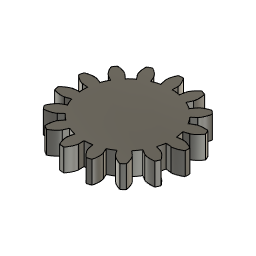
GearTrain v2 (Autodesk Fusion 360 archive; units mm, degrees)
design "15T Mod 2 Gear Base"
Autodesk Fusion 360 part; units mm, degrees
(part 1 of 2)
sketch "Sketch1" plane through (0, 0, 0) normal (0, 0, 1) x (1, 0, 0) in component "Component"
  spline S0 degree 5 poles (13.996, -1.6823) (13.9961, -1.6823) (13.9965, -1.6823) (13.9971, -1.6824) (13.998, -1.6825) (13.9993, -1.6826) (14.0009, -1.6828) (14.0027, -1.6829) (14.0047, -1.6831) (14.0069, -1.6833) (14.0093, -1.6834) (14.0119, -1.6836) (14.0147, -1.6838) (14.0177, -1.684) (14.0209, -1.6842) (14.0242, -1.6844) (14.0278, -1.6846) (14.0315, -1.6848) (14.0354, -1.6849) (14.0394, -1.6851) (14.0436, -1.6853) (14.048, -1.6854) (14.0525, -1.6856) (14.0572, -1.6857) (14.0621, -1.6858) (14.0671, -1.6859) (14.0723, -1.686) (14.0776, -1.6861) (14.083, -1.6861) (14.0886, -1.6861) (14.0944, -1.6862) (14.1003, -1.6861) (14.1063, -1.6861) (14.1124, -1.6861) (14.1187, -1.686) (14.1252, -1.6859) (14.1317, -1.6858) (14.1384, -1.6856) (14.1453, -1.6855) (14.1522, -1.6853) (14.1593, -1.685) (14.1665, -1.6848) (14.1738, -1.6845) (14.1812, -1.6842) (14.1888, -1.6839) (14.1965, -1.6835) (14.2042, -1.6831) (14.2122, -1.6827) (14.2202, -1.6822) (14.2283, -1.6817) (14.2365, -1.6812) (14.2449, -1.6806) (14.2533, -1.68) (14.2619, -1.6794) (14.2706, -1.6787) (14.2794, -1.678) (14.2882, -1.6773) (14.2972, -1.6765) (14.3063, -1.6757) (14.3155, -1.6748) (14.3248, -1.674) (14.3341, -1.673) (14.3436, -1.6721) (14.3532, -1.6711) (14.3629, -1.67) (14.3726, -1.6689) (14.3825, -1.6678) (14.3924, -1.6666) (14.4024, -1.6654) (14.4126, -1.6642) (14.4228, -1.6629) (14.4331, -1.6616) (14.4435, -1.6602) (14.4539, -1.6588) (14.4645, -1.6573) (14.4752, -1.6558) (14.4859, -1.6542) (14.4967, -1.6527) (14.5076, -1.651) (14.5186, -1.6493) (14.5296, -1.6476) (14.5408, -1.6458) (14.552, -1.644) (14.5633, -1.6421) (14.5746, -1.6402) (14.5861, -1.6383) (14.5976, -1.6363) (14.6092, -1.6342) (14.6209, -1.6321) (14.6326, -1.63) (14.6444, -1.6278) (14.6563, -1.6255) (14.6683, -1.6233) (14.6803, -1.6209) (14.6924, -1.6185) (14.7046, -1.6161) (14.7168, -1.6136) (14.7292, -1.6111) (14.7415, -1.6085) (14.754, -1.6059) (14.7665, -1.6032) (14.7791, -1.6004) (14.7917, -1.5977) (14.8044, -1.5948) (14.8172, -1.5919) (14.83, -1.589) (14.8429, -1.586) (14.8559, -1.583) (14.8689, -1.5799) (14.882, -1.5767) (14.8951, -1.5735) (14.9083, -1.5703) (14.9216, -1.567) (14.9349, -1.5636) (14.9483, -1.5602) (14.9617, -1.5568) (14.9752, -1.5533) (14.9888, -1.5497) (15.0024, -1.5461) (15.0161, -1.5424) (15.0298, -1.5387) (15.0435, -1.5349) (15.0574, -1.5311) (15.0713, -1.5272) (15.0852, -1.5233) (15.0992, -1.5193) (15.1132, -1.5152) (15.1273, -1.5111) (15.1414, -1.507) (15.1556, -1.5028) (15.1699, -1.4985) (15.1842, -1.4942) (15.1985, -1.4898) (15.2129, -1.4854) (15.2273, -1.4809) (15.2418, -1.4764) (15.2563, -1.4718) (15.2709, -1.4671) (15.2855, -1.4624) (15.3002, -1.4577) (15.3149, -1.4529) (15.3297, -1.448) (15.3445, -1.443) (15.3594, -1.4381) (15.3743, -1.433) (15.3892, -1.4279) (15.4042, -1.4228) (15.4192, -1.4176) (15.4343, -1.4123) (15.4494, -1.407) (15.4645, -1.4016) (15.4797, -1.3962) (15.4949, -1.3907) (15.5102, -1.3851) (15.5255, -1.3795) (15.5409, -1.3738) (15.5563, -1.3681) (15.5717, -1.3623) (15.5871, -1.3565) (15.6027, -1.3506) (15.6182, -1.3446) (15.6338, -1.3386) (15.6494, -1.3326) (15.665, -1.3264) (15.6807, -1.3202) (15.6964, -1.314) (15.7122, -1.3077) (15.728, -1.3014) (15.7438, -1.2949) (15.7597, -1.2885) (15.7756, -1.2819) (15.7915, -1.2753) (15.8075, -1.2687) (15.8234, -1.262) (15.8395, -1.2552) (15.8555, -1.2484) (15.8716, -1.2415) (15.8877, -1.2346) (15.9039, -1.2276) (15.9201, -1.2205) (15.9363, -1.2134) (15.9525, -1.2062) (15.9688, -1.199) (15.9851, -1.1917) (16.0014, -1.1843) (16.0178, -1.1769) (16.0342, -1.1695) (16.0506, -1.1619) (16.067, -1.1543) (16.0835, -1.1467) (16.1, -1.139) (16.1165, -1.1312) (16.133, -1.1234) (16.1496, -1.1155) (16.1662, -1.1076) (16.1828, -1.0996) (16.1995, -1.0915) (16.2162, -1.0834) (16.2329, -1.0752) (16.2496, -1.067) (16.2663, -1.0587) (16.2831, -1.0503) (16.2999, -1.0419) (16.3167, -1.0334) (16.3336, -1.0249) (16.3504, -1.0163) (16.3673, -1.0076) (16.3842, -0.9989) (16.4011, -0.9901) (16.4181, -0.9813) (16.435, -0.9724) (16.452, -0.9635) (16.469, -0.9544) (16.4861, -0.9454) (16.5031, -0.9362) (16.5202, -0.927) (16.5373, -0.9178) (16.5544, -0.9085) (16.5715, -0.8991) (16.5886, -0.8897) (16.6058, -0.8802) (16.623, -0.8706) (16.6402, -0.861) (16.6574, -0.8513) (16.6746, -0.8416) (16.6919, -0.8318) (16.7091, -0.822) (16.7264, -0.8121) (16.7437, -0.8021) (16.761, -0.7921) (16.7783, -0.782) (16.7957, -0.7718) (16.813, -0.7616) (16.8304, -0.7514) (16.8478, -0.741) (16.8652, -0.7306) (16.8826, -0.7202) (16.9, -0.7097) (16.9174, -0.6991) (16.9349, -0.6885) (16.9524, -0.6778) (16.9663, -0.6692) (16.9768, -0.6627) (16.9838, -0.6584) (16.9873, -0.6562) knots 0 0 0 0 0 0 0.00416667 0.00833333 0.0125 0.01666667 0.02083333 0.025 0.02916667 0.03333333 0.0375 0.04166667 0.04583333 0.05 0.05416667 0.05833333 0.0625 0.06666667 0.07083333 0.075 0.07916667 0.08333333 0.0875 0.09166667 0.09583333 0.1 0.10416667 0.10833333 0.1125 0.11666667 0.12083333 0.125 0.12916667 0.13333333 0.1375 0.14166667 0.14583333 0.15 0.15416667 0.15833333 0.1625 0.16666667 0.17083333 0.175 0.17916667 0.18333333 0.1875 0.19166667 0.19583333 0.2 0.20416667 0.20833333 0.2125 0.21666667 0.22083333 0.225 0.22916667 0.23333333 0.2375 0.24166667 0.24583333 0.25 0.25416667 0.25833333 0.2625 0.26666667 0.27083333 0.275 0.27916667 0.28333333 0.2875 0.29166667 0.29583333 0.3 0.30416667 0.30833333 0.3125 0.31666667 0.32083333 0.325 0.32916667 0.33333333 0.3375 0.34166667 0.34583333 0.35 0.35416667 0.35833333 0.3625 0.36666667 0.37083333 0.375 0.37916667 0.38333333 0.3875 0.39166667 0.39583333 0.4 0.40416667 0.40833333 0.4125 0.41666667 0.42083333 0.425 0.42916667 0.43333333 0.4375 0.44166667 0.44583333 0.45 0.45416667 0.45833333 0.4625 0.46666667 0.47083333 0.475 0.47916667 0.48333333 0.4875 0.49166667 0.49583333 0.5 0.50416667 0.50833333 0.5125 0.51666667 0.52083333 0.525 0.52916667 0.53333333 0.5375 0.54166667 0.54583333 0.55 0.55416667 0.55833333 0.5625 0.56666667 0.57083333 0.575 0.57916667 0.58333333 0.5875 0.59166667 0.59583333 0.6 0.60416667 0.60833333 0.6125 0.61666667 0.62083333 0.625 0.62916667 0.63333333 0.6375 0.64166667 0.64583333 0.65 0.65416667 0.65833333 0.6625 0.66666667 0.67083333 0.675 0.67916667 0.68333333 0.6875 0.69166667 0.69583333 0.7 0.70416667 0.70833333 0.7125 0.71666667 0.72083333 0.725 0.72916667 0.73333333 0.7375 0.74166667 0.74583333 0.75 0.75416667 0.75833333 0.7625 0.76666667 0.77083333 0.775 0.77916667 0.78333333 0.7875 0.79166667 0.79583333 0.8 0.80416667 0.80833333 0.8125 0.81666667 0.82083333 0.825 0.82916667 0.83333333 0.8375 0.84166667 0.84583333 0.85 0.85416667 0.85833333 0.8625 0.86666667 0.87083333 0.875 0.87916667 0.88333333 0.8875 0.89166667 0.89583333 0.9 0.90416667 0.90833333 0.9125 0.91666667 0.92083333 0.925 0.92916667 0.93333333 0.9375 0.94166667 0.94583333 0.95 0.95416667 0.95833333 0.9625 0.96666667 0.97083333 0.975 0.97916667 0.98333333 0.9875 0.99166667 0.99583333 1 1 1 1 1 1
  spline S1 degree 5 poles (13.996, 1.6823) (13.9961, 1.6823) (13.9965, 1.6823) (13.9971, 1.6824) (13.998, 1.6825) (13.9993, 1.6826) (14.0009, 1.6828) (14.0027, 1.6829) (14.0047, 1.6831) (14.0069, 1.6833) (14.0093, 1.6834) (14.0119, 1.6836) (14.0147, 1.6838) (14.0177, 1.684) (14.0209, 1.6842) (14.0242, 1.6844) (14.0278, 1.6846) (14.0315, 1.6848) (14.0354, 1.6849) (14.0394, 1.6851) (14.0436, 1.6853) (14.048, 1.6854) (14.0525, 1.6856) (14.0572, 1.6857) (14.0621, 1.6858) (14.0671, 1.6859) (14.0723, 1.686) (14.0776, 1.6861) (14.083, 1.6861) (14.0886, 1.6861) (14.0944, 1.6862) (14.1003, 1.6861) (14.1063, 1.6861) (14.1124, 1.6861) (14.1187, 1.686) (14.1252, 1.6859) (14.1317, 1.6858) (14.1384, 1.6856) (14.1453, 1.6855) (14.1522, 1.6853) (14.1593, 1.685) (14.1665, 1.6848) (14.1738, 1.6845) (14.1812, 1.6842) (14.1888, 1.6839) (14.1965, 1.6835) (14.2042, 1.6831) (14.2122, 1.6827) (14.2202, 1.6822) (14.2283, 1.6817) (14.2365, 1.6812) (14.2449, 1.6806) (14.2533, 1.68) (14.2619, 1.6794) (14.2706, 1.6787) (14.2794, 1.678) (14.2882, 1.6773) (14.2972, 1.6765) (14.3063, 1.6757) (14.3155, 1.6748) (14.3248, 1.674) (14.3341, 1.673) (14.3436, 1.6721) (14.3532, 1.6711) (14.3629, 1.67) (14.3726, 1.6689) (14.3825, 1.6678) (14.3924, 1.6666) (14.4024, 1.6654) (14.4126, 1.6642) (14.4228, 1.6629) (14.4331, 1.6616) (14.4435, 1.6602) (14.4539, 1.6588) (14.4645, 1.6573) (14.4752, 1.6558) (14.4859, 1.6542) (14.4967, 1.6527) (14.5076, 1.651) (14.5186, 1.6493) (14.5296, 1.6476) (14.5408, 1.6458) (14.552, 1.644) (14.5633, 1.6421) (14.5746, 1.6402) (14.5861, 1.6383) (14.5976, 1.6363) (14.6092, 1.6342) (14.6209, 1.6321) (14.6326, 1.63) (14.6444, 1.6278) (14.6563, 1.6255) (14.6683, 1.6233) (14.6803, 1.6209) (14.6924, 1.6185) (14.7046, 1.6161) (14.7168, 1.6136) (14.7292, 1.6111) (14.7415, 1.6085) (14.754, 1.6059) (14.7665, 1.6032) (14.7791, 1.6004) (14.7917, 1.5977) (14.8044, 1.5948) (14.8172, 1.5919) (14.83, 1.589) (14.8429, 1.586) (14.8559, 1.583) (14.8689, 1.5799) (14.882, 1.5767) (14.8951, 1.5735) (14.9083, 1.5703) (14.9216, 1.567) (14.9349, 1.5636) (14.9483, 1.5602) (14.9617, 1.5568) (14.9752, 1.5533) (14.9888, 1.5497) (15.0024, 1.5461) (15.0161, 1.5424) (15.0298, 1.5387) (15.0435, 1.5349) (15.0574, 1.5311) (15.0713, 1.5272) (15.0852, 1.5233) (15.0992, 1.5193) (15.1132, 1.5152) (15.1273, 1.5111) (15.1414, 1.507) (15.1556, 1.5028) (15.1699, 1.4985) (15.1842, 1.4942) (15.1985, 1.4898) (15.2129, 1.4854) (15.2273, 1.4809) (15.2418, 1.4764) (15.2563, 1.4718) (15.2709, 1.4671) (15.2855, 1.4624) (15.3002, 1.4577) (15.3149, 1.4529) (15.3297, 1.448) (15.3445, 1.443) (15.3594, 1.4381) (15.3743, 1.433) (15.3892, 1.4279) (15.4042, 1.4228) (15.4192, 1.4176) (15.4343, 1.4123) (15.4494, 1.407) (15.4645, 1.4016) (15.4797, 1.3962) (15.4949, 1.3907) (15.5102, 1.3851) (15.5255, 1.3795) (15.5409, 1.3738) (15.5563, 1.3681) (15.5717, 1.3623) (15.5871, 1.3565) (15.6027, 1.3506) (15.6182, 1.3446) (15.6338, 1.3386) (15.6494, 1.3326) (15.665, 1.3264) (15.6807, 1.3202) (15.6964, 1.314) (15.7122, 1.3077) (15.728, 1.3014) (15.7438, 1.2949) (15.7597, 1.2885) (15.7756, 1.2819) (15.7915, 1.2753) (15.8075, 1.2687) (15.8234, 1.262) (15.8395, 1.2552) (15.8555, 1.2484) (15.8716, 1.2415) (15.8877, 1.2346) (15.9039, 1.2276) (15.9201, 1.2205) (15.9363, 1.2134) (15.9525, 1.2062) (15.9688, 1.199) (15.9851, 1.1917) (16.0014, 1.1843) (16.0178, 1.1769) (16.0342, 1.1695) (16.0506, 1.1619) (16.067, 1.1543) (16.0835, 1.1467) (16.1, 1.139) (16.1165, 1.1312) (16.133, 1.1234) (16.1496, 1.1155) (16.1662, 1.1076) (16.1828, 1.0996) (16.1995, 1.0915) (16.2162, 1.0834) (16.2329, 1.0752) (16.2496, 1.067) (16.2663, 1.0587) (16.2831, 1.0503) (16.2999, 1.0419) (16.3167, 1.0334) (16.3336, 1.0249) (16.3504, 1.0163) (16.3673, 1.0076) (16.3842, 0.9989) (16.4011, 0.9901) (16.4181, 0.9813) (16.435, 0.9724) (16.452, 0.9635) (16.469, 0.9544) (16.4861, 0.9454) (16.5031, 0.9362) (16.5202, 0.927) (16.5373, 0.9178) (16.5544, 0.9085) (16.5715, 0.8991) (16.5886, 0.8897) (16.6058, 0.8802) (16.623, 0.8706) (16.6402, 0.861) (16.6574, 0.8513) (16.6746, 0.8416) (16.6919, 0.8318) (16.7091, 0.822) (16.7264, 0.8121) (16.7437, 0.8021) (16.761, 0.7921) (16.7783, 0.782) (16.7957, 0.7718) (16.813, 0.7616) (16.8304, 0.7514) (16.8478, 0.741) (16.8652, 0.7306) (16.8826, 0.7202) (16.9, 0.7097) (16.9174, 0.6991) (16.9349, 0.6885) (16.9524, 0.6778) (16.9663, 0.6692) (16.9768, 0.6627) (16.9838, 0.6584) (16.9873, 0.6562) knots 0 0 0 0 0 0 0.00416667 0.00833333 0.0125 0.01666667 0.02083333 0.025 0.02916667 0.03333333 0.0375 0.04166667 0.04583333 0.05 0.05416667 0.05833333 0.0625 0.06666667 0.07083333 0.075 0.07916667 0.08333333 0.0875 0.09166667 0.09583333 0.1 0.10416667 0.10833333 0.1125 0.11666667 0.12083333 0.125 0.12916667 0.13333333 0.1375 0.14166667 0.14583333 0.15 0.15416667 0.15833333 0.1625 0.16666667 0.17083333 0.175 0.17916667 0.18333333 0.1875 0.19166667 0.19583333 0.2 0.20416667 0.20833333 0.2125 0.21666667 0.22083333 0.225 0.22916667 0.23333333 0.2375 0.24166667 0.24583333 0.25 0.25416667 0.25833333 0.2625 0.26666667 0.27083333 0.275 0.27916667 0.28333333 0.2875 0.29166667 0.29583333 0.3 0.30416667 0.30833333 0.3125 0.31666667 0.32083333 0.325 0.32916667 0.33333333 0.3375 0.34166667 0.34583333 0.35 0.35416667 0.35833333 0.3625 0.36666667 0.37083333 0.375 0.37916667 0.38333333 0.3875 0.39166667 0.39583333 0.4 0.40416667 0.40833333 0.4125 0.41666667 0.42083333 0.425 0.42916667 0.43333333 0.4375 0.44166667 0.44583333 0.45 0.45416667 0.45833333 0.4625 0.46666667 0.47083333 0.475 0.47916667 0.48333333 0.4875 0.49166667 0.49583333 0.5 0.50416667 0.50833333 0.5125 0.51666667 0.52083333 0.525 0.52916667 0.53333333 0.5375 0.54166667 0.54583333 0.55 0.55416667 0.55833333 0.5625 0.56666667 0.57083333 0.575 0.57916667 0.58333333 0.5875 0.59166667 0.59583333 0.6 0.60416667 0.60833333 0.6125 0.61666667 0.62083333 0.625 0.62916667 0.63333333 0.6375 0.64166667 0.64583333 0.65 0.65416667 0.65833333 0.6625 0.66666667 0.67083333 0.675 0.67916667 0.68333333 0.6875 0.69166667 0.69583333 0.7 0.70416667 0.70833333 0.7125 0.71666667 0.72083333 0.725 0.72916667 0.73333333 0.7375 0.74166667 0.74583333 0.75 0.75416667 0.75833333 0.7625 0.76666667 0.77083333 0.775 0.77916667 0.78333333 0.7875 0.79166667 0.79583333 0.8 0.80416667 0.80833333 0.8125 0.81666667 0.82083333 0.825 0.82916667 0.83333333 0.8375 0.84166667 0.84583333 0.85 0.85416667 0.85833333 0.8625 0.86666667 0.87083333 0.875 0.87916667 0.88333333 0.8875 0.89166667 0.89583333 0.9 0.90416667 0.90833333 0.9125 0.91666667 0.92083333 0.925 0.92916667 0.93333333 0.9375 0.94166667 0.94583333 0.95 0.95416667 0.95833333 0.9625 0.96666667 0.97083333 0.975 0.97916667 0.98333333 0.9875 0.99166667 0.99583333 1 1 1 1 1 1
  spline S2 degree 5 poles (13.9947, -1.6821) (13.9947, -1.6821) (13.9948, -1.6821) (13.995, -1.6822) (13.9952, -1.6822) (13.9955, -1.6822) (13.9957, -1.6822) (13.9958, -1.6823) (13.9959, -1.6823) (13.996, -1.6823) knots 0 0 0 0 0 0 0.2 0.4 0.6 0.8 1 1 1 1 1 1
  spline S3 degree 5 poles (13.9947, 1.6821) (13.9947, 1.6821) (13.9948, 1.6821) (13.995, 1.6822) (13.9952, 1.6822) (13.9955, 1.6822) (13.9957, 1.6822) (13.9958, 1.6823) (13.9959, 1.6823) (13.996, 1.6823) knots 0 0 0 0 0 0 0.2 0.4 0.6 0.8 1 1 1 1 1 1
  line L0 (0, 0) -> (13.9947, -1.6821)
  line L1 (0, 0) -> (13.9947, 1.6821)
  arc A0 (16.9873, -0.6562) -> (16.9873, 0.6562) centre (0, 0) ccw
  point P0 (14, -1.6827)
  point P1 (14.0066, -1.6832)
  point P2 (14.0159, -1.6839)
  point P3 (14.0279, -1.6846)
  point P4 (14.0426, -1.6852)
  point P5 (14.0599, -1.6858)
  point P6 (14.0799, -1.6861)
  point P7 (14.1026, -1.6861)
  point P8 (14.128, -1.6858)
  point P9 (14.156, -1.6851)
  point P10 (14.1867, -1.684)
  point P11 (14.22, -1.6822)
  point P12 (14.2559, -1.6798)
  point P13 (14.2945, -1.6767)
  point P14 (14.3357, -1.6729)
  point P15 (14.3795, -1.6681)
  point P16 (14.4258, -1.6625)
  point P17 (14.4747, -1.6558)
  point P18 (14.5262, -1.6481)
  point P19 (14.5802, -1.6393)
  point P20 (14.6367, -1.6292)
  point P21 (14.6957, -1.6179)
  point P22 (14.7571, -1.6052)
  point P23 (14.8209, -1.5911)
  point P24 (14.8872, -1.5755)
  point P25 (14.9558, -1.5583)
  point P26 (15.0267, -1.5395)
  point P27 (15.1, -1.5191)
  point P28 (15.1755, -1.4968)
  point P29 (15.2532, -1.4728)
  point P30 (15.3332, -1.4468)
  point P31 (15.4153, -1.4189)
  point P32 (15.4996, -1.389)
  point P33 (15.5859, -1.3569)
  point P34 (15.6743, -1.3228)
  point P35 (15.7646, -1.2864)
  point P36 (15.857, -1.2478)
  point P37 (15.9512, -1.2068)
  point P38 (16.0473, -1.1634)
  point P39 (16.1452, -1.1176)
  point P40 (16.2448, -1.0693)
  point P41 (16.3462, -1.0184)
  point P42 (16.4492, -0.9649)
  point P43 (16.5538, -0.9088)
  point P44 (16.66, -0.8498)
  point P45 (16.7677, -0.7882)
  point P46 (16.8768, -0.7236)
  point P47 (14, 1.6827)
  point P48 (14.0066, 1.6832)
  point P49 (14.0159, 1.6839)
  point P50 (14.0279, 1.6846)
  point P51 (14.0426, 1.6852)
  point P52 (14.0599, 1.6858)
  point P53 (14.0799, 1.6861)
  point P54 (14.1026, 1.6861)
  point P55 (14.128, 1.6858)
  point P56 (14.156, 1.6851)
  point P57 (14.1867, 1.684)
  point P58 (14.22, 1.6822)
  point P59 (14.2559, 1.6798)
  point P60 (14.2945, 1.6767)
  point P61 (14.3357, 1.6729)
  point P62 (14.3795, 1.6681)
  point P63 (14.4258, 1.6625)
  point P64 (14.4747, 1.6558)
  point P65 (14.5262, 1.6481)
  point P66 (14.5802, 1.6393)
  point P67 (14.6367, 1.6292)
  point P68 (14.6957, 1.6179)
  point P69 (14.7571, 1.6052)
  point P70 (14.8209, 1.5911)
  point P71 (14.8872, 1.5755)
  point P72 (14.9558, 1.5583)
  point P73 (15.0267, 1.5395)
  point P74 (15.1, 1.5191)
  point P75 (15.1755, 1.4968)
  point P76 (15.2532, 1.4728)
  point P77 (15.3332, 1.4468)
  point P78 (15.4153, 1.4189)
  point P79 (15.4996, 1.389)
  point P80 (15.5859, 1.3569)
  point P81 (15.6743, 1.3228)
  point P82 (15.7646, 1.2864)
  point P83 (15.857, 1.2478)
  point P84 (15.9512, 1.2068)
  point P85 (16.0473, 1.1634)
  point P86 (16.1452, 1.1176)
  point P87 (16.2448, 1.0693)
  point P88 (16.3462, 1.0184)
  point P89 (16.4492, 0.9649)
  point P90 (16.5538, 0.9088)
  point P91 (16.66, 0.8498)
  point P92 (16.7677, 0.7882)
  point P93 (16.8768, 0.7236)
sketch "Sketch2" plane through (0, 0, 0) normal (0, 0, 1) x (1, 0, 0) in component "Component"
  circle A0 centre (0, 0) radius 12.5
extrude "Extrude1" add sketch "Sketch2" along normal blind 6.35 makes body 1 in component "Component"
extrude "Extrude2" add sketch "Sketch1" along normal blind 6.35 separate body makes body 2 in component "Component"
pattern_circular "C-Pattern1" count 15 over 360 about axis through (0, 0, 1.75) along (0, 0, 1) of "Extrude2" makes body 3 at (4.4901, 1.3853, 2.1167) makes body 4 at (3.5384, 3.0918, 2.1167) makes body 5 at (0.9084, 4.6103, 2.1167) makes body 6 at (0.07, 4.6984, 2.1167) makes body 7 at (-2.8183, 3.7599, 2.1167) makes body 8 at (-3.4447, 3.1959, 2.1167) makes body 9 at (-4.4468, 1.5185, 2.1167) makes body 10 at (-4.68, -0.4215, 2.1167) makes body 11 at (-4.1039, -2.2885, 2.1167) makes body 12 at (-2.8183, -3.7599, 2.1167) makes body 13 at (0.07, -4.6984, 2.1167) makes body 14 at (1.975, -4.2637, 2.1167) makes body 15 at (3.5384, -3.0918, 2.1167) makes body 16 at (4.0339, -2.4098, 2.1167) in component "Component"
combine "Combine1" operation add target body 1 tool bodies 2 3 4 5 6 7 8 9 10 11 12 13 14 15 16 in component "Component"
sketch "Sketch3" plane through (0, 0, 0) normal (0, 0, 1) x (1, 0, 0) in component "Component"
  line L0 (0, 0) -> (50.8594, 0) construction
  line L1 (50.8594, 0) -> (50.8594, 3) construction
  line L2 (50.8594, 3) -> (0, 3) construction
  line L3 (0, 3) -> (0, 0) construction
  constraint perpendicular L0 L1
  constraint parallel L0 L2
  constraint parallel L1 L3
component "Component" placed x (1, 0, 0) y (0, 1, 0) z (0, 0, 1) at (0, 0, 0)

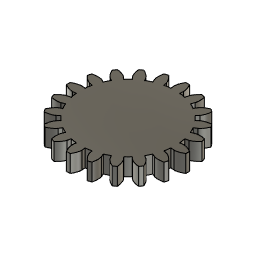
design "20T Mod 2 Gear"
Autodesk Fusion 360 part; units mm, degrees
sketch "Sketch1" plane through (0, 0, 0) normal (0, 0, 1) x (1, 0, 0) in component "Component"
  spline S0 degree 5 poles (18.7133, -1.7537) (18.7135, -1.7538) (18.7139, -1.7538) (18.7145, -1.7538) (18.7155, -1.7539) (18.7171, -1.754) (18.7188, -1.7541) (18.7208, -1.7543) (18.7231, -1.7544) (18.7256, -1.7546) (18.7283, -1.7547) (18.7312, -1.7548) (18.7343, -1.755) (18.7376, -1.7551) (18.7412, -1.7553) (18.7449, -1.7554) (18.7488, -1.7555) (18.753, -1.7557) (18.7573, -1.7558) (18.7618, -1.7559) (18.7665, -1.756) (18.7714, -1.756) (18.7764, -1.7561) (18.7816, -1.7561) (18.787, -1.7562) (18.7926, -1.7562) (18.7983, -1.7562) (18.8042, -1.7562) (18.8103, -1.7561) (18.8165, -1.756) (18.8228, -1.756) (18.8293, -1.7558) (18.836, -1.7557) (18.8428, -1.7556) (18.8498, -1.7554) (18.8569, -1.7552) (18.8641, -1.7549) (18.8715, -1.7547) (18.8791, -1.7544) (18.8867, -1.7541) (18.8945, -1.7537) (18.9025, -1.7533) (18.9105, -1.7529) (18.9187, -1.7525) (18.927, -1.752) (18.9355, -1.7515) (18.9441, -1.751) (18.9528, -1.7504) (18.9616, -1.7498) (18.9705, -1.7492) (18.9796, -1.7485) (18.9887, -1.7478) (18.998, -1.7471) (19.0074, -1.7463) (19.017, -1.7455) (19.0266, -1.7446) (19.0363, -1.7437) (19.0462, -1.7428) (19.0562, -1.7418) (19.0662, -1.7408) (19.0764, -1.7398) (19.0867, -1.7387) (19.0971, -1.7376) (19.1075, -1.7364) (19.1181, -1.7352) (19.1288, -1.7339) (19.1396, -1.7327) (19.1505, -1.7313) (19.1615, -1.73) (19.1726, -1.7285) (19.1837, -1.7271) (19.195, -1.7256) (19.2064, -1.724) (19.2178, -1.7225) (19.2294, -1.7208) (19.241, -1.7192) (19.2527, -1.7174) (19.2645, -1.7157) (19.2765, -1.7139) (19.2884, -1.712) (19.3005, -1.7101) (19.3127, -1.7082) (19.3249, -1.7062) (19.3373, -1.7041) (19.3497, -1.702) (19.3622, -1.6999) (19.3748, -1.6977) (19.3874, -1.6955) (19.4002, -1.6932) (19.413, -1.6909) (19.4259, -1.6885) (19.4389, -1.6861) (19.4519, -1.6836) (19.465, -1.6811) (19.4782, -1.6786) (19.4915, -1.6759) (19.5049, -1.6733) (19.5183, -1.6706) (19.5318, -1.6678) (19.5454, -1.665) (19.559, -1.6621) (19.5727, -1.6592) (19.5865, -1.6563) (19.6004, -1.6532) (19.6143, -1.6502) (19.6283, -1.6471) (19.6423, -1.6439) (19.6565, -1.6407) (19.6707, -1.6374) (19.6849, -1.6341) (19.6992, -1.6307) (19.7136, -1.6273) (19.7281, -1.6238) (19.7426, -1.6203) (19.7572, -1.6167) (19.7718, -1.6131) (19.7865, -1.6094) (19.8013, -1.6056) (19.8161, -1.6019) (19.831, -1.598) (19.846, -1.5941) (19.861, -1.5902) (19.876, -1.5862) (19.8912, -1.5821) (19.9063, -1.578) (19.9216, -1.5738) (19.9369, -1.5696) (19.9522, -1.5653) (19.9676, -1.561) (19.9831, -1.5566) (19.9986, -1.5522) (20.0142, -1.5477) (20.0298, -1.5431) (20.0455, -1.5385) (20.0612, -1.5339) (20.077, -1.5292) (20.0929, -1.5244) (20.1087, -1.5196) (20.1247, -1.5147) (20.1407, -1.5098) (20.1567, -1.5048) (20.1728, -1.4998) (20.1889, -1.4947) (20.2051, -1.4895) (20.2214, -1.4843) (20.2377, -1.4791) (20.254, -1.4737) (20.2704, -1.4684) (20.2868, -1.4629) (20.3033, -1.4574) (20.3198, -1.4519) (20.3364, -1.4463) (20.353, -1.4407) (20.3696, -1.4349) (20.3863, -1.4292) (20.4031, -1.4233) (20.4199, -1.4175) (20.4367, -1.4115) (20.4536, -1.4055) (20.4705, -1.3995) (20.4874, -1.3934) (20.5044, -1.3872) (20.5215, -1.381) (20.5385, -1.3747) (20.5557, -1.3684) (20.5728, -1.362) (20.59, -1.3555) (20.6073, -1.349) (20.6246, -1.3425) (20.6419, -1.3358) (20.6592, -1.3292) (20.6766, -1.3224) (20.6941, -1.3156) (20.7115, -1.3088) (20.729, -1.3019) (20.7466, -1.2949) (20.7642, -1.2879) (20.7818, -1.2808) (20.7994, -1.2736) (20.8171, -1.2664) (20.8348, -1.2592) (20.8526, -1.2519) (20.8704, -1.2445) (20.8882, -1.2371) (20.9061, -1.2296) (20.924, -1.222) (20.9419, -1.2144) (20.9598, -1.2067) (20.9778, -1.199) (20.9959, -1.1912) (21.0139, -1.1834) (21.032, -1.1755) (21.0501, -1.1676) (21.0683, -1.1595) (21.0864, -1.1515) (21.1046, -1.1433) (21.1229, -1.1351) (21.1411, -1.1269) (21.1594, -1.1186) (21.1778, -1.1102) (21.1961, -1.1018) (21.2145, -1.0933) (21.2329, -1.0848) (21.2513, -1.0762) (21.2698, -1.0675) (21.2883, -1.0588) (21.3068, -1.05) (21.3254, -1.0412) (21.3439, -1.0323) (21.3625, -1.0233) (21.3811, -1.0143) (21.3998, -1.0053) (21.4185, -0.9961) (21.4372, -0.9869) (21.4559, -0.9777) (21.4746, -0.9684) (21.4934, -0.959) (21.5122, -0.9496) (21.531, -0.9401) (21.5499, -0.9306) (21.5687, -0.921) (21.5876, -0.9113) (21.6065, -0.9016) (21.6255, -0.8918) (21.6444, -0.882) (21.6634, -0.8721) (21.6824, -0.8621) (21.7014, -0.8521) (21.7204, -0.842) (21.7395, -0.8319) (21.7586, -0.8217) (21.7777, -0.8114) (21.7968, -0.8011) (21.8159, -0.7908) (21.8351, -0.7803) (21.8543, -0.7699) (21.8735, -0.7593) (21.8927, -0.7487) (21.9119, -0.738) (21.9312, -0.7273) (21.9504, -0.7165) (21.9659, -0.7078) (21.9774, -0.7013) (21.9852, -0.697) (21.989, -0.6948) knots 0 0 0 0 0 0 0.00416667 0.00833333 0.0125 0.01666667 0.02083333 0.025 0.02916667 0.03333333 0.0375 0.04166667 0.04583333 0.05 0.05416667 0.05833333 0.0625 0.06666667 0.07083333 0.075 0.07916667 0.08333333 0.0875 0.09166667 0.09583333 0.1 0.10416667 0.10833333 0.1125 0.11666667 0.12083333 0.125 0.12916667 0.13333333 0.1375 0.14166667 0.14583333 0.15 0.15416667 0.15833333 0.1625 0.16666667 0.17083333 0.175 0.17916667 0.18333333 0.1875 0.19166667 0.19583333 0.2 0.20416667 0.20833333 0.2125 0.21666667 0.22083333 0.225 0.22916667 0.23333333 0.2375 0.24166667 0.24583333 0.25 0.25416667 0.25833333 0.2625 0.26666667 0.27083333 0.275 0.27916667 0.28333333 0.2875 0.29166667 0.29583333 0.3 0.30416667 0.30833333 0.3125 0.31666667 0.32083333 0.325 0.32916667 0.33333333 0.3375 0.34166667 0.34583333 0.35 0.35416667 0.35833333 0.3625 0.36666667 0.37083333 0.375 0.37916667 0.38333333 0.3875 0.39166667 0.39583333 0.4 0.40416667 0.40833333 0.4125 0.41666667 0.42083333 0.425 0.42916667 0.43333333 0.4375 0.44166667 0.44583333 0.45 0.45416667 0.45833333 0.4625 0.46666667 0.47083333 0.475 0.47916667 0.48333333 0.4875 0.49166667 0.49583333 0.5 0.50416667 0.50833333 0.5125 0.51666667 0.52083333 0.525 0.52916667 0.53333333 0.5375 0.54166667 0.54583333 0.55 0.55416667 0.55833333 0.5625 0.56666667 0.57083333 0.575 0.57916667 0.58333333 0.5875 0.59166667 0.59583333 0.6 0.60416667 0.60833333 0.6125 0.61666667 0.62083333 0.625 0.62916667 0.63333333 0.6375 0.64166667 0.64583333 0.65 0.65416667 0.65833333 0.6625 0.66666667 0.67083333 0.675 0.67916667 0.68333333 0.6875 0.69166667 0.69583333 0.7 0.70416667 0.70833333 0.7125 0.71666667 0.72083333 0.725 0.72916667 0.73333333 0.7375 0.74166667 0.74583333 0.75 0.75416667 0.75833333 0.7625 0.76666667 0.77083333 0.775 0.77916667 0.78333333 0.7875 0.79166667 0.79583333 0.8 0.80416667 0.80833333 0.8125 0.81666667 0.82083333 0.825 0.82916667 0.83333333 0.8375 0.84166667 0.84583333 0.85 0.85416667 0.85833333 0.8625 0.86666667 0.87083333 0.875 0.87916667 0.88333333 0.8875 0.89166667 0.89583333 0.9 0.90416667 0.90833333 0.9125 0.91666667 0.92083333 0.925 0.92916667 0.93333333 0.9375 0.94166667 0.94583333 0.95 0.95416667 0.95833333 0.9625 0.96666667 0.97083333 0.975 0.97916667 0.98333333 0.9875 0.99166667 0.99583333 1 1 1 1 1 1
  spline S1 degree 5 poles (18.7133, 1.7537) (18.7135, 1.7538) (18.7139, 1.7538) (18.7145, 1.7538) (18.7155, 1.7539) (18.7171, 1.754) (18.7188, 1.7541) (18.7208, 1.7543) (18.7231, 1.7544) (18.7256, 1.7546) (18.7283, 1.7547) (18.7312, 1.7548) (18.7343, 1.755) (18.7376, 1.7551) (18.7412, 1.7553) (18.7449, 1.7554) (18.7488, 1.7555) (18.753, 1.7557) (18.7573, 1.7558) (18.7618, 1.7559) (18.7665, 1.756) (18.7714, 1.756) (18.7764, 1.7561) (18.7816, 1.7561) (18.787, 1.7562) (18.7926, 1.7562) (18.7983, 1.7562) (18.8042, 1.7562) (18.8103, 1.7561) (18.8165, 1.756) (18.8228, 1.756) (18.8293, 1.7558) (18.836, 1.7557) (18.8428, 1.7556) (18.8498, 1.7554) (18.8569, 1.7552) (18.8641, 1.7549) (18.8715, 1.7547) (18.8791, 1.7544) (18.8867, 1.7541) (18.8945, 1.7537) (18.9025, 1.7533) (18.9105, 1.7529) (18.9187, 1.7525) (18.927, 1.752) (18.9355, 1.7515) (18.9441, 1.751) (18.9528, 1.7504) (18.9616, 1.7498) (18.9705, 1.7492) (18.9796, 1.7485) (18.9887, 1.7478) (18.998, 1.7471) (19.0074, 1.7463) (19.017, 1.7455) (19.0266, 1.7446) (19.0363, 1.7437) (19.0462, 1.7428) (19.0562, 1.7418) (19.0662, 1.7408) (19.0764, 1.7398) (19.0867, 1.7387) (19.0971, 1.7376) (19.1075, 1.7364) (19.1181, 1.7352) (19.1288, 1.7339) (19.1396, 1.7327) (19.1505, 1.7313) (19.1615, 1.73) (19.1726, 1.7285) (19.1837, 1.7271) (19.195, 1.7256) (19.2064, 1.724) (19.2178, 1.7225) (19.2294, 1.7208) (19.241, 1.7192) (19.2527, 1.7174) (19.2645, 1.7157) (19.2765, 1.7139) (19.2884, 1.712) (19.3005, 1.7101) (19.3127, 1.7082) (19.3249, 1.7062) (19.3373, 1.7041) (19.3497, 1.702) (19.3622, 1.6999) (19.3748, 1.6977) (19.3874, 1.6955) (19.4002, 1.6932) (19.413, 1.6909) (19.4259, 1.6885) (19.4389, 1.6861) (19.4519, 1.6836) (19.465, 1.6811) (19.4782, 1.6786) (19.4915, 1.6759) (19.5049, 1.6733) (19.5183, 1.6706) (19.5318, 1.6678) (19.5454, 1.665) (19.559, 1.6621) (19.5727, 1.6592) (19.5865, 1.6563) (19.6004, 1.6532) (19.6143, 1.6502) (19.6283, 1.6471) (19.6423, 1.6439) (19.6565, 1.6407) (19.6707, 1.6374) (19.6849, 1.6341) (19.6992, 1.6307) (19.7136, 1.6273) (19.7281, 1.6238) (19.7426, 1.6203) (19.7572, 1.6167) (19.7718, 1.6131) (19.7865, 1.6094) (19.8013, 1.6056) (19.8161, 1.6019) (19.831, 1.598) (19.846, 1.5941) (19.861, 1.5902) (19.876, 1.5862) (19.8912, 1.5821) (19.9063, 1.578) (19.9216, 1.5738) (19.9369, 1.5696) (19.9522, 1.5653) (19.9676, 1.561) (19.9831, 1.5566) (19.9986, 1.5522) (20.0142, 1.5477) (20.0298, 1.5431) (20.0455, 1.5385) (20.0612, 1.5339) (20.077, 1.5292) (20.0929, 1.5244) (20.1087, 1.5196) (20.1247, 1.5147) (20.1407, 1.5098) (20.1567, 1.5048) (20.1728, 1.4998) (20.1889, 1.4947) (20.2051, 1.4895) (20.2214, 1.4843) (20.2377, 1.4791) (20.254, 1.4737) (20.2704, 1.4684) (20.2868, 1.4629) (20.3033, 1.4574) (20.3198, 1.4519) (20.3364, 1.4463) (20.353, 1.4407) (20.3696, 1.4349) (20.3863, 1.4292) (20.4031, 1.4233) (20.4199, 1.4175) (20.4367, 1.4115) (20.4536, 1.4055) (20.4705, 1.3995) (20.4874, 1.3934) (20.5044, 1.3872) (20.5215, 1.381) (20.5385, 1.3747) (20.5557, 1.3684) (20.5728, 1.362) (20.59, 1.3555) (20.6073, 1.349) (20.6246, 1.3425) (20.6419, 1.3358) (20.6592, 1.3292) (20.6766, 1.3224) (20.6941, 1.3156) (20.7115, 1.3088) (20.729, 1.3019) (20.7466, 1.2949) (20.7642, 1.2879) (20.7818, 1.2808) (20.7994, 1.2736) (20.8171, 1.2664) (20.8348, 1.2592) (20.8526, 1.2519) (20.8704, 1.2445) (20.8882, 1.2371) (20.9061, 1.2296) (20.924, 1.222) (20.9419, 1.2144) (20.9598, 1.2067) (20.9778, 1.199) (20.9959, 1.1912) (21.0139, 1.1834) (21.032, 1.1755) (21.0501, 1.1676) (21.0683, 1.1595) (21.0864, 1.1515) (21.1046, 1.1433) (21.1229, 1.1351) (21.1411, 1.1269) (21.1594, 1.1186) (21.1778, 1.1102) (21.1961, 1.1018) (21.2145, 1.0933) (21.2329, 1.0848) (21.2513, 1.0762) (21.2698, 1.0675) (21.2883, 1.0588) (21.3068, 1.05) (21.3254, 1.0412) (21.3439, 1.0323) (21.3625, 1.0233) (21.3811, 1.0143) (21.3998, 1.0053) (21.4185, 0.9961) (21.4372, 0.9869) (21.4559, 0.9777) (21.4746, 0.9684) (21.4934, 0.959) (21.5122, 0.9496) (21.531, 0.9401) (21.5499, 0.9306) (21.5687, 0.921) (21.5876, 0.9113) (21.6065, 0.9016) (21.6255, 0.8918) (21.6444, 0.882) (21.6634, 0.8721) (21.6824, 0.8621) (21.7014, 0.8521) (21.7204, 0.842) (21.7395, 0.8319) (21.7586, 0.8217) (21.7777, 0.8114) (21.7968, 0.8011) (21.8159, 0.7908) (21.8351, 0.7803) (21.8543, 0.7699) (21.8735, 0.7593) (21.8927, 0.7487) (21.9119, 0.738) (21.9312, 0.7273) (21.9504, 0.7165) (21.9659, 0.7078) (21.9774, 0.7013) (21.9852, 0.697) (21.989, 0.6948) knots 0 0 0 0 0 0 0.00416667 0.00833333 0.0125 0.01666667 0.02083333 0.025 0.02916667 0.03333333 0.0375 0.04166667 0.04583333 0.05 0.05416667 0.05833333 0.0625 0.06666667 0.07083333 0.075 0.07916667 0.08333333 0.0875 0.09166667 0.09583333 0.1 0.10416667 0.10833333 0.1125 0.11666667 0.12083333 0.125 0.12916667 0.13333333 0.1375 0.14166667 0.14583333 0.15 0.15416667 0.15833333 0.1625 0.16666667 0.17083333 0.175 0.17916667 0.18333333 0.1875 0.19166667 0.19583333 0.2 0.20416667 0.20833333 0.2125 0.21666667 0.22083333 0.225 0.22916667 0.23333333 0.2375 0.24166667 0.24583333 0.25 0.25416667 0.25833333 0.2625 0.26666667 0.27083333 0.275 0.27916667 0.28333333 0.2875 0.29166667 0.29583333 0.3 0.30416667 0.30833333 0.3125 0.31666667 0.32083333 0.325 0.32916667 0.33333333 0.3375 0.34166667 0.34583333 0.35 0.35416667 0.35833333 0.3625 0.36666667 0.37083333 0.375 0.37916667 0.38333333 0.3875 0.39166667 0.39583333 0.4 0.40416667 0.40833333 0.4125 0.41666667 0.42083333 0.425 0.42916667 0.43333333 0.4375 0.44166667 0.44583333 0.45 0.45416667 0.45833333 0.4625 0.46666667 0.47083333 0.475 0.47916667 0.48333333 0.4875 0.49166667 0.49583333 0.5 0.50416667 0.50833333 0.5125 0.51666667 0.52083333 0.525 0.52916667 0.53333333 0.5375 0.54166667 0.54583333 0.55 0.55416667 0.55833333 0.5625 0.56666667 0.57083333 0.575 0.57916667 0.58333333 0.5875 0.59166667 0.59583333 0.6 0.60416667 0.60833333 0.6125 0.61666667 0.62083333 0.625 0.62916667 0.63333333 0.6375 0.64166667 0.64583333 0.65 0.65416667 0.65833333 0.6625 0.66666667 0.67083333 0.675 0.67916667 0.68333333 0.6875 0.69166667 0.69583333 0.7 0.70416667 0.70833333 0.7125 0.71666667 0.72083333 0.725 0.72916667 0.73333333 0.7375 0.74166667 0.74583333 0.75 0.75416667 0.75833333 0.7625 0.76666667 0.77083333 0.775 0.77916667 0.78333333 0.7875 0.79166667 0.79583333 0.8 0.80416667 0.80833333 0.8125 0.81666667 0.82083333 0.825 0.82916667 0.83333333 0.8375 0.84166667 0.84583333 0.85 0.85416667 0.85833333 0.8625 0.86666667 0.87083333 0.875 0.87916667 0.88333333 0.8875 0.89166667 0.89583333 0.9 0.90416667 0.90833333 0.9125 0.91666667 0.92083333 0.925 0.92916667 0.93333333 0.9375 0.94166667 0.94583333 0.95 0.95416667 0.95833333 0.9625 0.96666667 0.97083333 0.975 0.97916667 0.98333333 0.9875 0.99166667 0.99583333 1 1 1 1 1 1
  spline S2 degree 5 poles (18.7119, -1.7536) (18.7119, -1.7536) (18.712, -1.7536) (18.7122, -1.7537) (18.7124, -1.7537) (18.7127, -1.7537) (18.713, -1.7537) (18.7131, -1.7537) (18.7132, -1.7537) (18.7133, -1.7537) knots 0 0 0 0 0 0 0.2 0.4 0.6 0.8 1 1 1 1 1 1
  spline S3 degree 5 poles (18.7119, 1.7536) (18.7119, 1.7536) (18.712, 1.7536) (18.7122, 1.7537) (18.7124, 1.7537) (18.7127, 1.7537) (18.713, 1.7537) (18.7131, 1.7537) (18.7132, 1.7537) (18.7133, 1.7537) knots 0 0 0 0 0 0 0.2 0.4 0.6 0.8 1 1 1 1 1 1
  line L0 (0, 0) -> (18.7119, -1.7536)
  line L1 (0, 0) -> (18.7119, 1.7536)
  arc A0 (21.989, -0.6948) -> (21.989, 0.6948) centre (0, 0) ccw
  point P0 (18.7176, -1.7541)
  point P1 (18.7249, -1.7545)
  point P2 (18.735, -1.755)
  point P3 (18.748, -1.7555)
  point P4 (18.764, -1.7559)
  point P5 (18.7828, -1.7561)
  point P6 (18.8046, -1.7561)
  point P7 (18.8292, -1.7558)
  point P8 (18.8567, -1.7552)
  point P9 (18.8871, -1.754)
  point P10 (18.9204, -1.7524)
  point P11 (18.9566, -1.7501)
  point P12 (18.9956, -1.7472)
  point P13 (19.0375, -1.7436)
  point P14 (19.0822, -1.7392)
  point P15 (19.1297, -1.7338)
  point P16 (19.18, -1.7276)
  point P17 (19.2332, -1.7203)
  point P18 (19.2891, -1.7119)
  point P19 (19.3477, -1.7024)
  point P20 (19.4091, -1.6916)
  point P21 (19.4732, -1.6795)
  point P22 (19.54, -1.6661)
  point P23 (19.6094, -1.6512)
  point P24 (19.6815, -1.6349)
  point P25 (19.7562, -1.6169)
  point P26 (19.8334, -1.5974)
  point P27 (19.9132, -1.5761)
  point P28 (19.9956, -1.553)
  point P29 (20.0804, -1.5282)
  point P30 (20.1677, -1.5014)
  point P31 (20.2574, -1.4726)
  point P32 (20.3495, -1.4418)
  point P33 (20.4439, -1.409)
  point P34 (20.5407, -1.3739)
  point P35 (20.6397, -1.3367)
  point P36 (20.7409, -1.2971)
  point P37 (20.8444, -1.2552)
  point P38 (20.9499, -1.211)
  point P39 (21.0576, -1.1642)
  point P40 (21.1674, -1.115)
  point P41 (21.2791, -1.0631)
  point P42 (21.3928, -1.0086)
  point P43 (21.5084, -0.9515)
  point P44 (21.6259, -0.8916)
  point P45 (21.7452, -0.8288)
  point P46 (21.8663, -0.7633)
  point P47 (18.7176, 1.7541)
  point P48 (18.7249, 1.7545)
  point P49 (18.735, 1.755)
  point P50 (18.748, 1.7555)
  point P51 (18.764, 1.7559)
  point P52 (18.7828, 1.7561)
  point P53 (18.8046, 1.7561)
  point P54 (18.8292, 1.7558)
  point P55 (18.8567, 1.7552)
  point P56 (18.8871, 1.754)
  point P57 (18.9204, 1.7524)
  point P58 (18.9566, 1.7501)
  point P59 (18.9956, 1.7472)
  point P60 (19.0375, 1.7436)
  point P61 (19.0822, 1.7392)
  point P62 (19.1297, 1.7338)
  point P63 (19.18, 1.7276)
  point P64 (19.2332, 1.7203)
  point P65 (19.2891, 1.7119)
  point P66 (19.3477, 1.7024)
  point P67 (19.4091, 1.6916)
  point P68 (19.4732, 1.6795)
  point P69 (19.54, 1.6661)
  point P70 (19.6094, 1.6512)
  point P71 (19.6815, 1.6349)
  point P72 (19.7562, 1.6169)
  point P73 (19.8334, 1.5974)
  point P74 (19.9132, 1.5761)
  point P75 (19.9956, 1.553)
  point P76 (20.0804, 1.5282)
  point P77 (20.1677, 1.5014)
  point P78 (20.2574, 1.4726)
  point P79 (20.3495, 1.4418)
  point P80 (20.4439, 1.409)
  point P81 (20.5407, 1.3739)
  point P82 (20.6397, 1.3367)
  point P83 (20.7409, 1.2971)
  point P84 (20.8444, 1.2552)
  point P85 (20.9499, 1.211)
  point P86 (21.0576, 1.1642)
  point P87 (21.1674, 1.115)
  point P88 (21.2791, 1.0631)
  point P89 (21.3928, 1.0086)
  point P90 (21.5084, 0.9515)
  point P91 (21.6259, 0.8916)
  point P92 (21.7452, 0.8288)
  point P93 (21.8663, 0.7633)
sketch "Sketch2" plane through (0, 0, 0) normal (0, 0, 1) x (1, 0, 0) in component "Component"
  circle A0 centre (0, 0) radius 17.5
extrude "Extrude1" add sketch "Sketch2" along normal blind 6.35 makes body 1 in component "Component"
extrude "Extrude2" add sketch "Sketch1" along normal blind 6.35 separate body makes body 2 in component "Component"
pattern_circular "C-Pattern1" count 20 over 360 about axis through (0, 0, 1.75) along (0, 0, 1) of "Extrude2" makes body 3 at (6.1131, 1.3716, 2.1167) makes body 4 at (4.7029, 4.1394, 2.1167) makes body 5 at (8.2788, 9.4057, 4.2333) makes body 6 at (2.4835, 5.7518, 2.1167) makes body 7 at (0.5846, 6.2378, 4.2333) makes body 8 at (-1.3716, 6.1131, 2.1167) makes body 9 at (-4.1394, 4.7029, 2.1167) makes body 10 at (-4.7029, 4.1394, 2.1167) makes body 11 at (-6.1131, 1.3716, 2.1167) makes body 12 at (-6.2378, 0.5846, 4.2333) makes body 13 at (-6.1131, -1.3716, 2.1167) makes body 14 at (-5.3901, -3.1935, 2.1167) makes body 15 at (-3.1935, -5.3901, 2.1167) makes body 16 at (-2.4835, -5.7518, 2.1167) makes body 17 at (-0.5846, -6.2378, 4.2333) makes body 18 at (1.3716, -6.1131, 2.1167) makes body 19 at (3.1935, -5.3901, 2.1167) makes body 20 at (4.7029, -4.1394, 2.1167) makes body 21 at (5.7518, -2.4835, 2.1167) in component "Component"
combine "Combine1" operation add target body 1 tool bodies 2 3 4 5 6 7 8 9 10 11 12 13 14 15 16 17 18 19 20 21 in component "Component"
sketch "Sketch3" plane through (0, 0, 0) normal (0, 0, 1) x (1, 0, 0) in component "Component"
  line L0 (0, 0) -> (50.8022, 0) construction
  line L1 (50.8022, 0) -> (50.8022, 3) construction
  line L2 (50.8022, 3) -> (0, 3) construction
  line L3 (0, 3) -> (0, 0) construction
  constraint perpendicular L0 L1
  constraint parallel L0 L2
  constraint parallel L1 L3
component "Component" placed x (1, 0, 0) y (0, 1, 0) z (0, 0, 1) at (0, 0, 0)

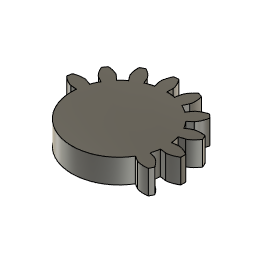
design "15T Mod 2 Slipgear"
Autodesk Fusion 360 part; units mm, degrees